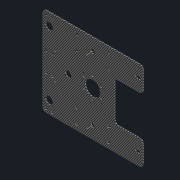
# Autodesk Inventor part: carbon_plate14
Saved by Autodesk Inventor 2021 (Build 250183000, 183)
## iProperties
Created: 2021-08-06
Part Number: carbon_plate14
Material: CFRP
Document SubType Name: Sheet Metal
Designer: yuta0
Density: 1.43 g/cm^3
Sheet Metal Rule: Default_mm
Appearance: カーボンファイバー
Mass: 58.4557 g
Surface Area: 430.885 cm^2
Volume: 40.8781 cm^3
購入先: カーボン
在庫数: 0.0
Author: yuta0
Autodesk Inventor part; units mm, degrees
ref_plane "YZ Plane" through (0, 0, 0) normal (1, 0, 0) x (0, 1, 0)
ref_plane "XZ Plane" through (0, 0, 0) normal (0, 1, 0) x (-1, 0, 0)
ref_plane "XY Plane" through (0, 0, 0) normal (0, 0, 1) x (1, 0, 0)
sketch "スケッチ1" plane through (0, 0, 0) normal (0, 0, 1) x (1, 0, 0)
  line L0 (-78, -69) -> (78, -69)
  line L1 (78, -69) -> (78, 69)
  line L2 (78, 69) -> (-78, 69)
  line L3 (-78, 69) -> (-78, -69)
  line L4 (-78, -69) -> (78, 69) construction
  line L5 (78, -69) -> (-78, 69) construction
  point P0 (0, 0)
  dimension "d0" = 156
  dimension "d1" = 138
  measures "d0" distance of L1.end L2.end
  measures "d1" distance of L2.end L0.start
extrude "プレート1" add sketch "スケッチ1" along normal blind 2
sketch "スケッチ2" plane through (0, 0, 2) normal (0, 0, 1) x (1, 0, 0)
  line L0 (-25, 39) -> (25, 39)
  line L1 (25, 39) -> (25, 61)
  line L2 (25, 61) -> (-25, 61)
  line L3 (-25, 61) -> (-25, 39)
  line L4 (-25, 39) -> (25, 61) construction
  line L5 (25, 39) -> (-25, 61) construction
  line L6 (-78, 69) -> (78, 69) projected
  point P0 (0, 0)
  point P1 (0, 50)
  point P2 (0, 50)
  point P3 (0, 50)
  dimension "d3" = 50
  dimension "d4" = 22
  dimension "d60" = 50
  constraints: 12 end point, 4 midpoint, 2 parallel, 1 horizontal, 1 perpendicular, 1 vertical alignment
  measures "d3" distance of L1.end L2.end
  measures "d4" distance of L2.end L0.start
  measures "d60" distance of point (0, 0) point (0, 50)
hole "穴1" at (-25, 61, 2) at (-25, 39, 2) at (25, 39, 2) at (25, 61, 2) direction (0, 0, -1) diameter 4.3 depth 2 clearance for "Flat Head Machine Screw" size "M4" standard "Ansi Metric M Profile"
sketch "スケッチ3" plane through (0, 0, 2) normal (0, 0, 1) x (1, 0, 0)
  line L0 (-63, 15.4) -> (-73, 15.4)
  line L1 (-73, 15.4) -> (-73, 64)
  line L2 (-73, 64) -> (-63, 64)
  line L3 (-63, 64) -> (-63, 15.4)
  line L4 (-63, 15.4) -> (-73, 64) construction
  line L5 (-73, 15.4) -> (-63, 64) construction
  line L6 (-78, 69) -> (78, 69) projected
  line L7 (-78, -69) -> (-78, 69) projected
  circle A0 centre (-68, 50) radius 6
  point P0 (0, 0)
  point P1 (-68, 39.7)
  point P2 (-68, 39.7)
  dimension "d18" = 10
  dimension "d19" = 48.6
  dimension "d20" = 14
  dimension "d31" = 19
  dimension "d47" = 68
  dimension "d48" = 12
  constraints: 12 end point, 3 midpoint, 2 parallel, 1 centre point, 1 coincident, 1 horizontal, 1 perpendicular, 1 vertical alignment
  measures "d18" distance of L1.end L2.end
  measures "d19" distance of L0.end L1.end
  measures "d20" distance from line of L2 point (-68, 50)
  measures "d31" distance from line of L6 point (-68, 50)
  measures "d47" horizontal distance of point (0, 0) point (-68, 50)
  measures "d48" diameter of A0
extrude "押し出し2" cut sketch "スケッチ3" against normal blind 10 contours A0 L1 L3 | L3 A0 | A0 L1
sketch "スケッチ7" plane through (0, 0, 2) normal (0, 0, 1) x (1, 0, 0)
  line L0 (68, 50) -> (73, 50) construction
  line L1 (68, 47.85) -> (73, 47.85)
  line L2 (73, 52.15) -> (68, 52.15)
  arc A0 (68, 52.15) -> (68, 47.85) centre (68, 50) ccw
  arc A1 (73, 47.85) -> (73, 52.15) centre (73, 50) ccw
  circle A2 centre (-68, 50) radius 6 projected
  point P0 (0, 0)
  point P1 (70.5, 50)
  dimension "d54" = 2.15
  dimension "d55" = 5
  dimension "d57" = 68
  constraints: 8 end point, 4 point on circle, 4 tangent, 2 centre point, 2 horizontal alignment, 1 midpoint, 1 parallel
  measures "d54" radius of A1
  measures "d55" distance of L0.start L0.end
  measures "d57" horizontal distance of point (0, 0) L0.start
extrude "押し出し3" cut sketch "スケッチ7" against normal blind 10 contours A0 L2 A1 L1
hole "穴2" at (-63, 15.4, 2) at (-73, 15.4, 2) at (-73, 64, 2) at (-63, 64, 2) direction (0, 0, -1) diameter 4.3 depth 2 clearance for "Flat Head Machine Screw" size "M4" standard "Ansi Metric M Profile"
sketch "スケッチ4" plane through (0, 0, 2) normal (0, 0, 1) x (1, 0, 0)
  circle A0 centre (0, 0) radius 16
  point P0 (0, 16)
  point P1 (-13.8564, 8)
  point P2 (-13.8564, -8)
  point P3 (0, -16)
  point P4 (13.8564, -8)
  point P5 (13.8564, 8)
  dimension "d32" = 32
  dimension "d35" = 360
  constraints: 1 coincident, 1 vertical alignment, 9 other
hole "穴3" at (0, 16, 2) at (-13.8564, 8, 2) at (-13.8564, -8, 2) at (0, -16, 2) at (13.8564, -8, 2) at (13.8564, 8, 2) direction (0, 0, -1) diameter 3.2 end through all clearance for "Socket Head Cap Screw" size "M3" standard "Ansi Metric M Profile"
sketch "スケッチ6" plane through (0, 0, 2) normal (0, 0, 1) x (1, 0, 0)
  point P0 (0, 0)
sketch "スケッチ8" plane through (0, 0, 0) normal (0, 0, -1) x (-1, 0, 0)
  point P0 (0, 0)
fillet "コーナーR1" radius 5 4 edges at (-78, 69, 1) (78, 69, 1) (78, -69, 1) (-78, -69, 1)
sketch "スケッチ10" plane through (0, 0, 2) normal (0, 0, 1) x (1, 0, 0)
  line L0 (-14, -14) -> (14, -14)
  line L1 (14, -14) -> (14, 14)
  line L2 (14, 14) -> (-14, 14)
  line L3 (-14, 14) -> (-14, -14)
  line L4 (-14, -14) -> (14, 14) construction
  line L5 (14, -14) -> (-14, 14) construction
  point P0 (0, 0)
  dimension "d70" = 28
  dimension "d71" = 28
  constraints: 12 end point, 2 midpoint, 2 parallel, 1 horizontal, 1 perpendicular
  measures "d70" distance of L2.end L1.end
  measures "d71" distance of L1.end L0.end
hole "穴4" at (14, 14, 2) at (-14, 14, 2) at (-14, -14, 2) at (14, -14, 2) direction (0, 0, -1) diameter 2.2 end through all clearance for "Flat Head Machine Screw" size "M2" standard "Ansi Metric M Profile"
sketch "スケッチ11" plane through (0, 0, 0) normal (0, 0, -1) x (-1, 0, 0)
  line L0 (-78, -64) -> (-78, 64) projected
  line L1 (78, -64) -> (78, 64) projected
  point P0 (0, 0)
  point P1 (58, -20.5)
  point P2 (58, 20.5)
  dimension "d79" = 41
  dimension "d92" = 20
  dimension "d93" = 20.5
  constraints: 1 vertical alignment
  measures "d79" distance of point (58, 20.5) point (58, -20.5)
  measures "d92" distance from line of L1 point (58, -20.5)
  measures "d93" vertical distance of point (0, 0) point (58, 20.5)
hole "穴5" at (-58, -20.5, 0) at (-58, 20.5, 0) direction (0, 0, 1) diameter 3.2 end through all clearance for "Flat Head Machine Screw" size "M3" standard "Ansi Metric M Profile"
sketch "スケッチ5" plane through (0, 0, 2) normal (0, 0, 1) x (1, 0, 0)
  circle A0 centre (0, 0) radius 12
  dimension "d44" = 24
  constraints: 1 centre point, 1 coincident
  measures "d44" diameter of A0
extrude "押し出し1" cut sketch "スケッチ5" against normal blind 10
sketch "スケッチ12" plane through (0, 0, 2) normal (0, 0, 1) x (1, 0, 0)
  point P0 (0, 0)
  point P1 (0, 50)
hole "穴6" at (0, 50, 2) direction (0, 0, -1) diameter 6 end through all
mirror "ミラー1" about plane through (0, 0, 0) normal (0, 1, 0) of "穴1", "押し出し2", "押し出し3", "穴2", "穴6"
sketch "スケッチ13" plane through (0, 0, 2) normal (0, 0, 1) x (1, 0, 0)
  circle A0 centre (-38, 0) radius 5
  point P0 (0, 0)
  dimension "d101" = 10
  dimension "d102" = 38
  constraints: 1 centre point, 1 horizontal alignment
  measures "d101" diameter of A0
  measures "d102" distance of point (0, 0) A0.centre
extrude "押し出し5" cut sketch "スケッチ13" against normal blind 10
sketch "スケッチ14" plane through (0, 0, 2) normal (0, 0, 1) x (1, 0, 0)
  line L0 (34, 31) -> (78, 31)
  line L1 (78, 31) -> (78, -31)
  line L2 (78, -31) -> (34, -31)
  line L3 (34, -31) -> (34, 31)
  line L4 (34, 31) -> (78, -31) construction
  line L5 (78, 31) -> (34, -31) construction
  line L6 (78, 64) -> (78, -64) projected
  line L7 (-73, 69) -> (73, 69) projected
  line L8 (73, -69) -> (-73, -69) projected
  point P0 (0, 0)
  point P1 (56, 0)
  dimension "d105" = 38
  dimension "d106" = 38
  dimension "d107" = 34
  constraints: 12 end point, 2 midpoint, 2 parallel, 1 horizontal, 1 perpendicular, 1 point on line
  measures "d105" distance between parallel lines of L7 L0
  measures "d106" distance between parallel lines of L8 L2
  measures "d107" distance from line of point (0, 0) L3
extrude "押し出し6" cut sketch "スケッチ14" against normal blind 10
fillet "コーナーR2" radius 5 4 edges at (78, 31, 1) (34, 31, 1) (34, -31, 1) (78, -31, 1)
equation "\"d14\" = Thickness"
equation "\"d28\" = Thickness"
equation "\"d42\" = Thickness"
equation "\"d77\" = Thickness"
equation "\"d93\" = 0.5 * d79"
equation "\"d88\" = Thickness"
equation "\"d99\" = Thickness"
equation "\"d2\" = Thickness"
equation "\"BendRadius\" = Thickness"
equation "\"BendReliefWidth\" = Thickness"
equation "\"BendReliefDepth\" = 0.5 * Thickness"
equation "\"CornerReliefSize\" = 4 * Thickness"
equation "\"MinimumRemnant\" = 2 * Thickness"
equation "\"TransitionRadius\" = BendRadius"
equation "\"JacobiRadiusSize\" = BendRadius"
equation "\"GapSize\" = Thickness"
equation "\"Thickness\" = 2"
